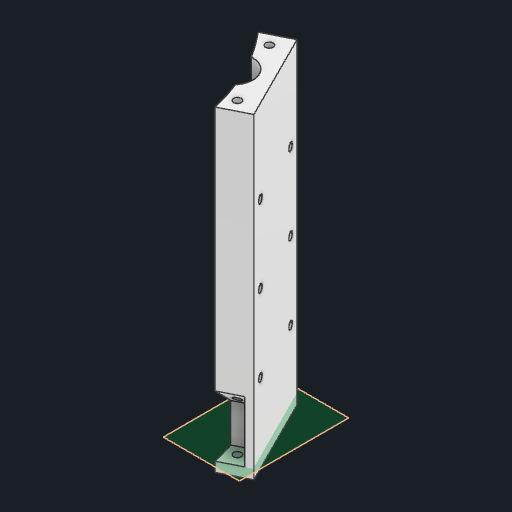
# Autodesk Inventor part: OUTK_024_SendHelp
Saved by Autodesk Inventor 2024.2 (Build 282272000, 272)
## iProperties
Created: 2024-12-08
Part Number: OUTK_024_SendHelp
Material: ABS Plastic
Document SubType Name: Modeling
Designer: Bryan
Density: 1.06 g/cm^3
Appearance: Smooth - White
Mass: 180.03 g
Surface Area: 442.833 cm^2
Volume: 169.839 cm^3
Author: Bryan
Autodesk Inventor part; units mm, degrees
ref_plane "YZ Plane" through (0, 0, 0) normal (1, 0, 0) x (0, 1, 0)
ref_plane "XZ Plane" through (0, 0, 0) normal (0, 1, 0) x (-1, 0, 0)
ref_plane "XY Plane" through (0, 0, 0) normal (0, 0, 1) x (1, 0, 0)
sketch "Sketch1" plane through (0, 0, 0) normal (0, 1, 0) x (-1, 0, 0)
  circle A0 centre (0, 0) radius 12.7
  arc A1 (1.0072, -12.66) -> (-9.5271, 8.3978) centre (114.5338, 57.2967) ccw projected
  arc A2 (1.0072, -12.66) -> (-9.5271, 8.3978) centre (114.5338, 57.2967) ccw projected
  spline S0 degree 3 poles (11.3039, -22.0073) (11.3199, -22.0281) (11.2645, -21.9561) (11.1207, -21.7683) (11.0008, -21.6114) (10.7243, -21.2473) (10.5484, -21.0146) (10.1658, -20.504) (9.9592, -20.2261) (9.5746, -19.7047) (9.3707, -19.4259) (8.997, -18.911) (8.8273, -18.6751) (8.562, -18.3045) (8.448, -18.1443) (8.2969, -17.9314) (8.2597, -17.8788) (8.2746, -17.8998) (8.2971, -17.9317) (8.4492, -18.146) (8.5639, -18.3072) (8.8299, -18.6787) (8.9993, -18.9142) (9.372, -19.4276) (9.5753, -19.7055) (9.9584, -20.225) (10.1641, -20.5018) (10.5454, -21.0107) (10.7208, -21.2428) (10.9982, -21.6081) (11.1191, -21.7662) (11.28, -21.9762) (11.3199, -22.0281) (11.3039, -22.0073) knots 0 0 0 0 0.095621 0.095621 0.191243 0.191243 0.288556 0.288556 0.385869 0.385869 0.482923 0.482923 0.579976 0.579976 0.675571 0.675571 0.771165 0.771165 0.86709 0.86709 0.963014 0.963014 1.059738 1.059738 1.156462 1.156462 1.253359 1.253359 1.350255 1.350255 1.446293 1.446293 1.542332 1.542332 1.542332 1.542332 projected
  spline S1 degree 3 poles (-9.3623, 17.3557) (-9.3544, 17.3312) (-9.3821, 17.4169) (-9.454, 17.641) (-9.5139, 17.8283) (-9.6513, 18.2629) (-9.7383, 18.5402) (-9.9262, 19.1479) (-10.027, 19.4783) (-10.2137, 20.0988) (-10.3122, 20.4307) (-10.4914, 21.0431) (-10.5722, 21.3234) (-10.6977, 21.763) (-10.7514, 21.9531) (-10.8224, 22.2058) (-10.8398, 22.2683) (-10.8328, 22.2433) (-10.8224, 22.2058) (-10.7514, 21.9531) (-10.6977, 21.763) (-10.5722, 21.3234) (-10.4914, 21.0431) (-10.3122, 20.4307) (-10.2137, 20.0988) (-10.027, 19.4783) (-9.9262, 19.1479) (-9.7383, 18.5402) (-9.6513, 18.2629) (-9.5139, 17.8283) (-9.454, 17.641) (-9.3742, 17.3924) (-9.3544, 17.3312) (-9.3623, 17.3557) knots 0 0 0 0 0.095595 0.095595 0.191189 0.191189 0.288243 0.288243 0.385297 0.385297 0.48261 0.48261 0.579923 0.579923 0.675544 0.675544 0.771165 0.771165 0.866787 0.866787 0.962408 0.962408 1.059721 1.059721 1.157034 1.157034 1.254088 1.254088 1.351142 1.351142 1.446736 1.446736 1.542331 1.542331 1.542331 1.542331 projected
  arc A3 (-9.5271, 8.3978) -> (1.0072, -12.66) centre (0, 0) ccw projected
  arc A4 (-15.5009, 27.7468) -> (-9.5271, 8.3978) centre (114.5338, 57.2967) ccw projected
  line L0 (-15.5009, 27.7468) -> (-32.538, 19.2238) projected
  line L1 (-32.538, 19.2238) -> (-4.1281, -37.5664) projected
  line L2 (-4.1281, -37.5664) -> (12.909, -29.0434) projected
  arc A5 (1.0072, -12.66) -> (12.909, -29.0434) centre (114.5338, 57.2967) ccw projected
  circle A6 centre (-19.192, 16.6381) radius 2.54 projected
  circle A7 centre (1.8059, -25.3357) radius 2.54 projected
  point P0 (11.3039, -22.0073)
  point P1 (-9.3623, 17.3557)
  dimension "d0" = 25.4
  constraints: 1 centre point, 1 coincident
  measures "d0" diameter of A0
extrude "Extrusion1" add sketch "Sketch1" along normal blind 207.9625 contours A0 A1 L2 L1 L0
sketch "Sketch2" plane through (4.1281, 0, -37.5664) normal (0.8943342, 0, -0.4473996) x (-0.4473996, 0, -0.8943342)
  spline S0 degree 3 poles (-51.435, 51.8428) (-51.435, 52.1625) (-51.4991, 52.5033) (-51.7587, 53.1291) (-51.9543, 53.4142) (-52.4055, 53.8654) (-52.6919, 54.0609) (-53.3178, 54.3196) (-53.6573, 54.3828) (-54.2932, 54.3828) (-54.6329, 54.3194) (-55.2586, 54.0606) (-55.5447, 53.8652) (-55.9954, 53.4144) (-56.191, 53.1296) (-56.4508, 52.5038) (-56.515, 52.1629) (-56.515, 51.5241) (-56.4513, 51.1845) (-56.1936, 50.5609) (-55.9996, 50.2767) (-55.5502, 49.8244) (-55.2634, 49.6276) (-54.6356, 49.3668) (-54.2946, 49.3028) (-53.6562, 49.3028) (-53.3157, 49.3664) (-52.6881, 49.6268) (-52.4011, 49.8234) (-51.951, 50.2758) (-51.7567, 50.5604) (-51.4987, 51.1845) (-51.435, 51.5241) (-51.435, 51.8428) knots 0 0 0 0 0.095924 0.095924 0.191848 0.191848 0.288573 0.288573 0.385297 0.385297 0.482193 0.482193 0.57909 0.57909 0.675128 0.675128 0.771166 0.771166 0.866788 0.866788 0.962409 0.962409 1.059722 1.059722 1.157035 1.157035 1.254089 1.254089 1.351143 1.351143 1.446737 1.446737 1.542332 1.542332 1.542332 1.542332 projected
  spline S1 degree 3 poles (-6.985, 51.8428) (-6.985, 52.1615) (-7.0487, 52.5011) (-7.3064, 53.1247) (-7.5004, 53.4089) (-7.9498, 53.8611) (-8.2366, 54.058) (-8.8644, 54.3188) (-9.2054, 54.3828) (-9.8438, 54.3828) (-10.1843, 54.3191) (-10.8119, 54.0588) (-11.0989, 53.8621) (-11.549, 53.4097) (-11.7433, 53.1252) (-12.0013, 52.5011) (-12.065, 52.1614) (-12.065, 51.5241) (-12.0013, 51.1845) (-11.7433, 50.5604) (-11.549, 50.2758) (-11.0989, 49.8234) (-10.8119, 49.6268) (-10.1843, 49.3664) (-9.8438, 49.3028) (-9.2054, 49.3028) (-8.8644, 49.3668) (-8.2366, 49.6276) (-7.9498, 49.8244) (-7.5004, 50.2767) (-7.3064, 50.5609) (-7.0487, 51.1845) (-6.985, 51.5241) (-6.985, 51.8428) knots 0 0 0 0 0.095621 0.095621 0.191243 0.191243 0.288556 0.288556 0.385869 0.385869 0.482923 0.482923 0.579976 0.579976 0.675571 0.675571 0.771165 0.771165 0.86676 0.86676 0.962355 0.962355 1.059408 1.059408 1.156462 1.156462 1.253775 1.253775 1.351088 1.351088 1.44671 1.44671 1.542331 1.542331 1.542331 1.542331 projected
  line L0 (0, 0) -> (-19.9771, 0) projected
  line L1 (-19.9771, 0) -> (-19.9771, 207.9625) projected
  line L2 (0, 207.9625) -> (-19.9771, 207.9625) projected
  line L3 (0, 0) -> (0, 207.9625) projected
  spline S2 degree 3 poles (-6.985, 102.6428) (-6.985, 102.9615) (-7.0487, 103.3011) (-7.3064, 103.9247) (-7.5004, 104.2089) (-7.9498, 104.6611) (-8.2366, 104.858) (-8.8644, 105.1188) (-9.2054, 105.1828) (-9.8438, 105.1828) (-10.1843, 105.1191) (-10.8119, 104.8588) (-11.0989, 104.6621) (-11.549, 104.2097) (-11.7433, 103.9252) (-12.0013, 103.3011) (-12.065, 102.9614) (-12.065, 102.323) (-12.0009, 101.9823) (-11.7413, 101.3565) (-11.5457, 101.0714) (-11.0945, 100.6202) (-10.8081, 100.4247) (-10.1822, 100.166) (-9.8427, 100.1028) (-9.2068, 100.1028) (-8.8671, 100.1662) (-8.2414, 100.425) (-7.9553, 100.6203) (-7.5046, 101.0711) (-7.309, 101.356) (-7.0492, 101.9817) (-6.985, 102.3227) (-6.985, 102.6428) knots 0 0 0 0 0.095621 0.095621 0.191243 0.191243 0.288556 0.288556 0.385869 0.385869 0.482923 0.482923 0.579976 0.579976 0.675571 0.675571 0.771165 0.771165 0.86709 0.86709 0.963014 0.963014 1.059738 1.059738 1.156462 1.156462 1.253359 1.253359 1.350255 1.350255 1.446293 1.446293 1.542332 1.542332 1.542332 1.542332 projected
  spline S3 degree 3 poles (-6.985, 153.4428) (-6.985, 153.7615) (-7.0487, 154.1011) (-7.3064, 154.7247) (-7.5004, 155.0089) (-7.9498, 155.4611) (-8.2366, 155.658) (-8.8644, 155.9188) (-9.2054, 155.9828) (-9.8438, 155.9828) (-10.1843, 155.9191) (-10.8119, 155.6588) (-11.0989, 155.4621) (-11.549, 155.0097) (-11.7433, 154.7252) (-12.0013, 154.1011) (-12.065, 153.7614) (-12.065, 153.123) (-12.0009, 152.7823) (-11.7413, 152.1565) (-11.5457, 151.8714) (-11.0945, 151.4202) (-10.8081, 151.2247) (-10.1822, 150.966) (-9.8427, 150.9028) (-9.2068, 150.9028) (-8.8671, 150.9662) (-8.2414, 151.225) (-7.9553, 151.4203) (-7.5046, 151.8711) (-7.309, 152.156) (-7.0492, 152.7817) (-6.985, 153.1227) (-6.985, 153.4428) knots 0 0 0 0 0.095621 0.095621 0.191243 0.191243 0.288556 0.288556 0.385869 0.385869 0.482923 0.482923 0.579976 0.579976 0.675571 0.675571 0.771165 0.771165 0.86709 0.86709 0.963014 0.963014 1.059738 1.059738 1.156462 1.156462 1.253359 1.253359 1.350255 1.350255 1.446293 1.446293 1.542332 1.542332 1.542332 1.542332 projected
  spline S4 degree 3 poles (-51.435, 102.6428) (-51.435, 102.9614) (-51.4987, 103.3011) (-51.7567, 103.9252) (-51.951, 104.2097) (-52.4011, 104.6621) (-52.6881, 104.8588) (-53.3157, 105.1191) (-53.6562, 105.1828) (-54.2946, 105.1828) (-54.6356, 105.1188) (-55.2634, 104.858) (-55.5502, 104.6611) (-55.9996, 104.2089) (-56.1936, 103.9247) (-56.4513, 103.3011) (-56.515, 102.9615) (-56.515, 102.3241) (-56.4513, 101.9845) (-56.1936, 101.3609) (-55.9996, 101.0767) (-55.5502, 100.6244) (-55.2634, 100.4276) (-54.6356, 100.1668) (-54.2946, 100.1028) (-53.6562, 100.1028) (-53.3157, 100.1664) (-52.6881, 100.4268) (-52.4011, 100.6234) (-51.951, 101.0758) (-51.7567, 101.3604) (-51.4987, 101.9845) (-51.435, 102.3241) (-51.435, 102.6428) knots 0 0 0 0 0.095595 0.095595 0.191189 0.191189 0.288243 0.288243 0.385297 0.385297 0.48261 0.48261 0.579923 0.579923 0.675544 0.675544 0.771165 0.771165 0.866787 0.866787 0.962408 0.962408 1.059721 1.059721 1.157034 1.157034 1.254088 1.254088 1.351142 1.351142 1.446736 1.446736 1.542331 1.542331 1.542331 1.542331 projected
  spline S5 degree 3 poles (-51.435, 153.4428) (-51.435, 153.7614) (-51.4987, 154.1011) (-51.7567, 154.7252) (-51.951, 155.0097) (-52.4011, 155.4621) (-52.6881, 155.6588) (-53.3157, 155.9191) (-53.6562, 155.9828) (-54.2946, 155.9828) (-54.6356, 155.9188) (-55.2634, 155.658) (-55.5502, 155.4611) (-55.9996, 155.0089) (-56.1936, 154.7247) (-56.4513, 154.1011) (-56.515, 153.7615) (-56.515, 153.1241) (-56.4513, 152.7845) (-56.1936, 152.1609) (-55.9996, 151.8767) (-55.5502, 151.4244) (-55.2634, 151.2276) (-54.6356, 150.9668) (-54.2946, 150.9028) (-53.6562, 150.9028) (-53.3157, 150.9664) (-52.6881, 151.2268) (-52.4011, 151.4234) (-51.951, 151.8758) (-51.7567, 152.1604) (-51.4987, 152.7845) (-51.435, 153.1241) (-51.435, 153.4428) knots 0 0 0 0 0.095595 0.095595 0.191189 0.191189 0.288243 0.288243 0.385297 0.385297 0.48261 0.48261 0.579923 0.579923 0.675544 0.675544 0.771165 0.771165 0.866787 0.866787 0.962408 0.962408 1.059721 1.059721 1.157034 1.157034 1.254088 1.254088 1.351142 1.351142 1.446736 1.446736 1.542331 1.542331 1.542331 1.542331 projected
  spline S6 degree 3 poles (-6.985, 153.4428) (-6.985, 153.7615) (-7.0487, 154.1011) (-7.3064, 154.7247) (-7.5004, 155.0089) (-7.9498, 155.4611) (-8.2366, 155.658) (-8.8644, 155.9188) (-9.2054, 155.9828) (-9.8438, 155.9828) (-10.1843, 155.9191) (-10.8119, 155.6588) (-11.0989, 155.4621) (-11.549, 155.0097) (-11.7433, 154.7252) (-12.0013, 154.1011) (-12.065, 153.7614) (-12.065, 153.123) (-12.0009, 152.7823) (-11.7413, 152.1565) (-11.5457, 151.8714) (-11.0945, 151.4202) (-10.8081, 151.2247) (-10.1822, 150.966) (-9.8427, 150.9028) (-9.2068, 150.9028) (-8.8671, 150.9662) (-8.2414, 151.225) (-7.9553, 151.4203) (-7.5046, 151.8711) (-7.309, 152.156) (-7.0492, 152.7817) (-6.985, 153.1227) (-6.985, 153.4428) knots 0 0 0 0 0.095621 0.095621 0.191243 0.191243 0.288556 0.288556 0.385869 0.385869 0.482923 0.482923 0.579976 0.579976 0.675571 0.675571 0.771165 0.771165 0.86709 0.86709 0.963014 0.963014 1.059738 1.059738 1.156462 1.156462 1.253359 1.253359 1.350255 1.350255 1.446293 1.446293 1.542332 1.542332 1.542332 1.542332 projected
  point P0 (-31.75, 0)
  point P1 (-51.435, 51.8428)
  point P2 (-6.985, 51.8428)
  point P3 (-6.985, 102.6428)
  point P4 (-6.985, 153.4428)
  point P5 (-51.435, 102.6428)
  point P6 (-51.435, 153.4428)
extrude "Extrusion2" cut sketch "Sketch2" against normal blind 188.9125 contours S0 | S1 | S2 | S3 | S4 | S5
ref_plane "Work Plane1" through (0, 6.35, 0) normal (0, -1, 0) x (1, 0, 0)
sketch "Sketch3" plane through (0, 6.35, 0) normal (0, -1, 0) x (1, 0, 0)
  circle A0 centre (-19.192, -16.6381) radius 2.54 projected
  circle A1 centre (19.192, 16.6381) radius 2.54 projected
  circle A2 centre (-1.8059, -25.3357) radius 2.54 projected
  circle A3 centre (1.8059, 25.3357) radius 2.54 projected
  circle A4 centre (0, 0) radius 12.7 projected
  arc A5 (15.5009, 27.7468) -> (-12.909, -29.0434) centre (-114.5338, 57.2967) ccw projected
  line L0 (-12.909, -29.0434) -> (4.1281, -37.5664) projected
  line L1 (4.1281, -37.5664) -> (32.538, 19.2238) projected
  line L2 (32.538, 19.2238) -> (15.5009, 27.7468) projected
  arc A6 (-12.909, -29.0434) -> (15.5009, 27.7468) centre (-114.5338, 57.2967) ccw
  line L3 (-3.9188, -17.1784) -> (6.7142, -22.4977)
  line L4 (6.7142, -22.4977) -> (0.1672, -35.5849)
  line L5 (11.397, 13.4374) -> (22.03, 8.1181)
  line L6 (22.03, 8.1181) -> (28.577, 21.2053)
  line L7 (32.538, 19.2238) -> (4.1281, -37.5664) projected
  point P0 (0, 0)
  dimension "d6" = 6.35
  dimension "d7" = 6.35
  constraints: 8 end point, 4 point on circle, 3 parallel, 2 equal length, 2 point on line, 1 centre point, 1 coincident, 1 perpendicular
  measures "d6" distance from line of A2.centre L3
  measures "d7" distance from line of L4 A2.centre
extrude "Extrusion3" cut sketch "Sketch3" against normal blind 25.4 contours A6 L2 L6 L5 | L3 L4 L0 A6
chamfer "Chamfer1" distance 14.605 angle 45 2 edges at (-6.3709, 31.75, -32.3142) (22.039, 31.75, 24.4761)
body "Solid1"
